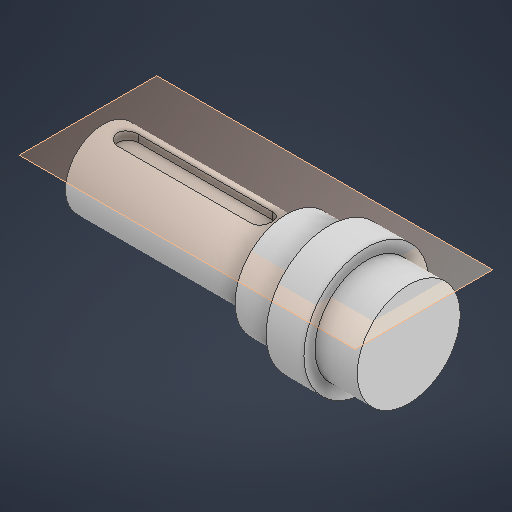
# Autodesk Inventor part: shaft_6
Saved by Autodesk Inventor 2026 (Build 300175050, 175E)
## iProperties
Created: 2025-09-24
Part Number: shaft_6
Material: Generisch
Document SubType Name: Modeling
Designer: tobia
Density: 1 g/cm^3
Appearance: Vorgabe
Author: tobia
Autodesk Inventor part; units mm, degrees
ref_plane "YZ Plane" through (0, 0, 0) normal (1, 0, 0) x (0, 1, 0)
ref_plane "XZ Plane" through (0, 0, 0) normal (0, 1, 0) x (-1, 0, 0)
sketch "Skizze1" plane through (0, 0, 0) normal (0, 0, 1) x (1, 0, 0)
  line L0 (0, 0) -> (0, 22)
  line L1 (0, 22) -> (107, 22)
  line L2 (107, 22) -> (107, 30)
  line L3 (107, 30) -> (131.65, 30)
  line L4 (131.65, 30) -> (131.65, 36.5)
  line L5 (131.65, 36.5) -> (153.65, 36.5)
  line L6 (153.65, 36.5) -> (153.65, 30)
  line L7 (153.65, 30) -> (178.3, 30)
  line L8 (178.3, 30) -> (178.3, 0)
  line L9 (178.3, 0) -> (0, 0)
  line L10 (-35.66, 0) -> (213.96, 0) projected
  constraints: 20 end point
revolve "Umdrehung1" add sketch "Skizze1" angle 360 about axis through (-10, 0, 0) along (1, 0, 0)
ref_plane "Arbeitsebene1" through (0, 0, 22) normal (0, 0, 1) x (1, 0, 0)
sketch "Skizze2" plane through (0, 0, 22) normal (0, 0, 1) x (1, 0, 0)
  line L0 (8.5, 0) -> (98.5, 0) construction
  line L1 (14.5, -6) -> (92.5, -6)
  line L2 (92.5, 6) -> (14.5, 6)
  arc A0 (14.5, 6) -> (14.5, -6) centre (14.5, 0) ccw
  arc A1 (92.5, -6) -> (92.5, 6) centre (92.5, 0) ccw
  point P0 (53.5, 0)
  constraints: 8 end point, 6 point on circle, 4 tangent, 2 centre point, 2 point on line, 1 midpoint, 1 parallel
extrude "Extrusion1" cut sketch "Skizze2" against normal blind 5
